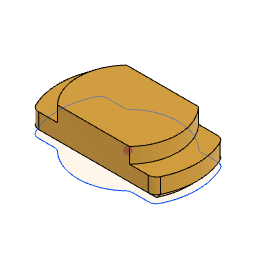
DiA Twist-Lock V2 20191026 (Autodesk Fusion 360 design; units mm, degrees)
Autodesk Fusion 360 part; units mm, degrees
sketch "Twist-Lock2 lock" plane through (0, 0, 0) normal (0, 0, 1) x (1, 0, 0)
  line L0 (7.7942, -4.5) -> (-7.7942, -4.5)
  line L1 (-7.7942, 4.5) -> (7.7942, 4.5)
  arc A0 (-7.7942, 4.5) -> (-7.7942, -4.5) centre (0, 0) ccw
  arc A1 (7.7942, -4.5) -> (7.7942, 4.5) centre (0, 0) ccw
  arc A2 (-4.6904, 4.5) -> (-4.6904, -4.5) centre (0, 0) ccw
  arc A3 (4.6904, -4.5) -> (4.6904, 4.5) centre (0, 0) ccw
  constraint coincident A0.centre A1.centre
  constraint parallel L0 L1
  constraint horizontal L0
  constraint coincident L1 A3.end
  constraint coincident L1 A2.start
  constraint concentric A0 A1
  constraint coincident L0 A2.end
  constraint coincident L0 A3.start
  constraint concentric A2 A3
sketch "Twist-Lock2 hole" plane through (0, 0, 0) normal (0, 0, 1) x (1, 0, 0)
  arc A0 (-8.093, 3.9375) -> (-8.093, -3.9375) centre (0, 0) ccw
  arc A1 (8.093, -3.9375) -> (8.093, 3.9375) centre (0, 0) ccw
  arc A2 (4.4192, 4.7667) -> (-4.4192, 4.7667) centre (0, 0) ccw
  arc A3 (-4.4192, -4.7667) -> (4.4192, -4.7667) centre (0, 0) ccw
  line L0 (7.1937, 4.5) -> (5.099, 4.5)
  line L1 (-5.099, 4.5) -> (-7.1937, 4.5)
  line L2 (-7.1937, -4.5) -> (-5.099, -4.5)
  line L3 (5.099, -4.5) -> (7.1937, -4.5)
  arc A4 (-5.099, 4.5) -> (-4.4192, 4.7667) centre (-5.099, 5.5) ccw
  arc A5 (-7.1937, 4.5) -> (-8.093, 3.9375) centre (-7.1937, 3.5) ccw
  arc A6 (-8.093, -3.9375) -> (-7.1937, -4.5) centre (-7.1937, -3.5) ccw
  arc A7 (-4.4192, -4.7667) -> (-5.099, -4.5) centre (-5.099, -5.5) ccw
  arc A8 (5.099, -4.5) -> (4.4192, -4.7667) centre (5.099, -5.5) ccw
  arc A9 (7.1937, -4.5) -> (8.093, -3.9375) centre (7.1937, -3.5) ccw
  arc A10 (8.093, 3.9375) -> (7.1937, 4.5) centre (7.1937, 3.5) ccw
  arc A11 (4.4192, 4.7667) -> (5.099, 4.5) centre (5.099, 5.5) ccw
  dimension "d26" = 1
  constraint coincident A0.centre A1.centre
  constraint parallel L0 L2
  constraint horizontal L0
  constraint concentric A0 A1
  constraint concentric A2 A3
  constraint collinear L0 L1
  constraint collinear L2 L3
  constraint tangent A2 A4
  constraint tangent L1 A4
  constraint tangent A0 A5
  constraint tangent L1 A5
  constraint equal A4 A5
  constraint tangent A0 A6
  constraint tangent L2 A6
  constraint equal A4 A6
  constraint tangent A3 A7
  constraint tangent L2 A7
  constraint equal A4 A7
  constraint tangent A3 A8
  constraint tangent L3 A8
  constraint equal A4 A8
  constraint tangent A1 A9
  constraint tangent L3 A9
  constraint equal A4 A9
  constraint tangent A1 A10
  constraint tangent L0 A10
  constraint equal A4 A10
  constraint tangent A2 A11
  constraint tangent L0 A11
  constraint equal A4 A11
  measures "d26" radius of A4
extrude "Extrude1" add sketch "Twist-Lock2 lock" along normal blind 3
extrude "Extrude2" add sketch "Twist-Lock2 lock" along normal blind 5 contours L0 L1 A2 A3
fillet "Fillet1" radius 1.1 4 edges at (7.7942, -4.5, 1.5) (-7.7942, -4.5, 1.5) (-7.7942, 4.5, 1.5) (7.7942, 4.5, 1.5)
chamfer "Chamfer1" distance 1 angle 45 8 edges at (-7.718, -4.3303, 0) (-9, 0, 0) (-7.718, 4.3303, 0) (0, 4.5, 0) (7.718, 4.3303, 0) (9, 0, 0) (7.718, -4.3303, 0) (0, -4.5, 0)
equation "Plate_thickness = 2 mm"
equation "Lock_thickness = 3 mm"
equation "d7 = Lock_thickness"
equation "d9 = Lock_thickness + Plate_thickness"
named bodies: "Twist-Lock2"
